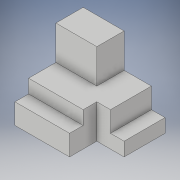
# Autodesk Inventor part: P3-2
Saved by Autodesk Inventor 2017 (Build 210142000, 142)
## iProperties
Created: 2017-02-10
Part Number: P3-2
Material: Generic
Document SubType Name: Modeling
Designer: Schaffel
Density: 1 g/cm^3
Appearance: Default
Author: Schaffel
Autodesk Inventor part; units mm, degrees
ref_plane "YZ Plane" through (0, 0, 0) normal (1, 0, 0) x (0, 1, 0)
ref_plane "XZ Plane" through (0, 0, 0) normal (0, 1, 0) x (-1, 0, 0)
ref_plane "XY Plane" through (0, 0, 0) normal (0, 0, 1) x (1, 0, 0)
sketch "Sketch1" plane through (0, 0, 0) normal (0, 0, 1) x (1, 0, 0)
  line L0 (0, 0) -> (76.2, 0)
  line L1 (76.2, 0) -> (76.2, 12.7)
  line L2 (76.2, 12.7) -> (63.5, 12.7)
  line L3 (63.5, 12.7) -> (63.5, 31.75)
  line L4 (63.5, 31.75) -> (38.1, 31.75)
  line L5 (38.1, 31.75) -> (38.1, 63.5)
  line L6 (38.1, 63.5) -> (0, 63.5)
  line L7 (0, 63.5) -> (0, 0)
  constraints: 16 end point, 7 perpendicular, 1 horizontal
extrude "Extrusion1" add sketch "Sketch1" along normal blind 25.4
sketch "Sketch2" plane through (0, 0, 25.4) normal (0, 0, 1) x (1, 0, 0)
  line L0 (63.5, 12.7) -> (63.5, 31.75) projected
  line L1 (63.5, 31.75) -> (0, 31.75)
  line L2 (63.5, 31.75) -> (38.1, 31.75) projected
  line L3 (0, 31.75) -> (0, 0)
  line L4 (0, 0) -> (76.2, 0) projected
  line L5 (0, 0) -> (76.2, 0)
  line L6 (76.2, 0) -> (76.2, 12.7) projected
  line L7 (76.2, 0) -> (76.2, 12.7)
  line L8 (76.2, 12.7) -> (63.5, 12.7) projected
  line L9 (76.2, 12.7) -> (63.5, 12.7)
  line L10 (63.5, 12.7) -> (63.5, 31.75)
  constraints: 12 end point, 4 collinear, 2 perpendicular
extrude "Extrusion2" add sketch "Sketch2" along normal blind 12.7
sketch "Sketch3" plane through (0, 0, 38.1) normal (0, 0, 1) x (1, 0, 0)
  line L0 (63.5, 31.75) -> (0, 31.75) projected
  line L1 (0, 31.75) -> (50.8, 31.75)
  line L2 (50.8, 0) -> (50.8, 31.75)
  line L3 (0, 0) -> (76.2, 0) projected
  line L4 (50.8, 0) -> (0, 0)
  line L5 (0, 31.75) -> (0, 0) projected
  line L6 (0, 0) -> (0, 31.75)
  constraints: 8 end point, 2 collinear, 1 perpendicular, 1 point on line
extrude "Extrusion3" add sketch "Sketch3" along normal blind 12.7
sketch "Sketch4" plane through (0, 0, 50.8) normal (0, 0, 1) x (1, 0, 0)
  line L0 (0, 0) -> (0, 19.05)
  line L1 (0, 63.5) -> (0, 0) projected
  line L2 (0, 19.05) -> (50.8, 19.05)
  line L3 (50.8, 31.75) -> (50.8, 0) projected
  line L4 (50.8, 19.05) -> (50.8, 0)
  line L5 (0, 0) -> (50.8, 0) projected
  line L6 (50.8, 0) -> (0, 0)
  constraints: 8 end point, 2 point on line, 1 collinear, 1 perpendicular, 1 vertical
extrude "Extrusion4" add sketch "Sketch4" along normal blind 12.7
body "Solid1"
